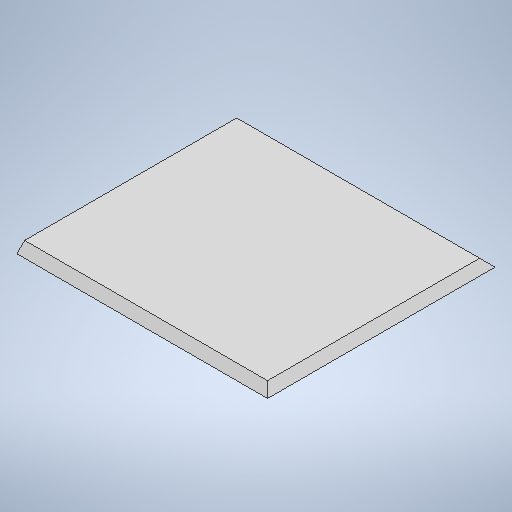
# Autodesk Inventor part: Part186
Saved by Autodesk Inventor 2025 (Build 290162000, 162)
## iProperties
Created: 2024-07-26
Part Number: Part186
Material: Generic
Document SubType Name: Modeling
Designer: Isaac
Density: 1 g/cm^3
Appearance: Default
Author: Isaac
Autodesk Inventor part; units mm, degrees
ref_plane "YZ Plane" through (0, 0, 0) normal (1, 0, 0) x (0, 1, 0)
ref_plane "XZ Plane" through (0, 0, 0) normal (0, 1, 0) x (-1, 0, 0)
ref_plane "XY Plane" through (0, 0, 0) normal (0, 0, 1) x (1, 0, 0)
sketch "Sketch1" plane through (0, 0, 0) normal (0, 1, 0) x (-1, 0, 0)
  line L0 (325, 295) -> (-325, 295)
  line L1 (-325, 295) -> (-325, -295)
  line L2 (-325, -295) -> (325, -295)
  line L3 (325, -295) -> (325, 295)
  line L4 (325, 295) -> (-325, -295) construction
  line L5 (-325, 295) -> (325, -295) construction
  point P0 (0, 0)
  dimension "d0" = 650
  dimension "d1" = 590
  constraints: 12 end point, 2 midpoint, 2 parallel, 1 horizontal, 1 perpendicular
  measures "d0" distance of L0.start L0.end
  measures "d1" distance of L2.end L0.start
extrude "Extrusion1" add sketch "Sketch1" along normal blind 20
chamfer "Chamfer3" distance 20 angle 45 3 edges at (0, 20, 295) (0, 20, -295) (325, 20, 0)
body "Solid1"
